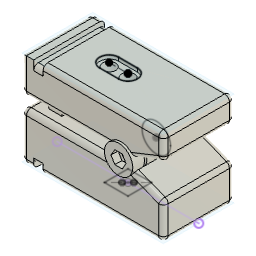
Pulse Oximeter v1 v4 (Autodesk Fusion 360 design; units mm, degrees)
Autodesk Fusion 360 part; units mm, degrees
sketch "Sketch1" plane through (0, 0, 0) normal (0, 0, 1) x (1, 0, 0)
  line L0 (30, 15) -> (-30, 15)
  line L1 (-30, 15) -> (-30, -15)
  line L2 (-30, -15) -> (30, -15)
  line L3 (30, -15) -> (30, 15)
  line L4 (30, 15) -> (-30, -15) construction
  line L5 (-30, 15) -> (30, -15) construction
  dimension "d1" = 30
  dimension "d2" = 60
  constraint horizontal L0
  constraint perpendicular L0 L1
  constraint parallel L0 L2
  constraint parallel L1 L3
  constraint coincident L4 origin
  constraint coincident L5 origin
  measures "d1" distance of L0 L2
  measures "d2" distance of L1 L3
extrude "Extrude1" add sketch "Sketch1" along normal blind 20 makes body 1
sketch "Sketch2" plane through (0, 0, 20) normal (0, 0, 1) x (-1, 0, 0)
  line L0 (-30, 15) -> (-30, -15)
  line L1 (-30, -15) -> (30, -15)
  line L2 (30, -15) -> (30, 15)
  line L3 (30, 15) -> (-30, 15)
  line L4 (30, -15) -> (-30, -15)
  line L5 (-30, -15) -> (-30, 15)
  line L6 (-30, 15) -> (30, 15)
  line L7 (30, 15) -> (30, -15)
  constraint horizontal L4
  constraint vertical L5
  constraint horizontal L6
  constraint vertical L7
  constraint coincident L0.start L3.end
  constraint coincident L1.end L2.start
extrude "Extrude2" add sketch "Sketch2" along normal blind 15 from surface at 5 separate body makes body 2
copy_body "Body->Comp1" bodies 2 removing the originals makes body 3 in component "Top"
sketch "Sketch3" plane through (0, 0, 0) normal (0, 1, 0) x (1, 0, 0)
  circle A0 centre (12, -22.5) radius 6
  line L0 (-30, 0) -> (30, 0)
  dimension "d8" = 12
  dimension "d9" = 12
  dimension "d10" = 22.5
  measures "d8" diameter of A0
  measures "d9" horizontal distance of origin A0.centre
  measures "d10" distance of A0.centre L0
move_face "MoveFace1" by (0, 0, 20) 1 faces at (10, 15, 30) on bodies 3 in component "Top"
move_body "Move1" bodies 1 to x (1, 0, 0) y (0, 1, 0) z (0, 0, 1) at (0, 0, -15)
extrude "Extrude1'" add sketch "Sketch3" along normal blind 5 from surface at 11 bodies 3 in component "Top"
extrude "Extrude2'" add sketch "Sketch3" along normal blind 5 from surface at -16 bodies 3 in component "Top"
sketch "Sketch4" plane through (0, 0, 0) normal (0, 1, 0) x (1, 0, 0)
  circle A0 centre (12, -7.5) radius 6
  line L0 (30, 15) -> (-30, 15)
  line L1 (30, 15) -> (30, -5)
  dimension "d17" = 12
  dimension "d19" = 22.5
  dimension "d20" = 18
  measures "d17" diameter of A0
  measures "d19" distance of A0.centre L0
  measures "d20" distance of A0.centre L1
extrude "Extrude3" add sketch "Sketch4" along normal mid plane 20 bodies 1
extrude "Extrude4" cut sketch "Sketch4" along normal through all from surface at 10 bodies 1
extrude "Extrude5" cut sketch "Sketch4" along normal up to surface (10 mm away) from surface at -20 bodies 1
move_body "Move2" bodies 1 to x (1, 0, 0) y (0, 1, 0) z (0, 0, 1) at (0, 0, 15)
sketch "Sketch5" plane through (0, 16, 0) normal (0, 1, 0) x (-1, 0, 0)
  circle A0 centre (-12, 22.5) radius 6
  circle A1 centre (-12, 22.5) radius 1.5
  dimension "d28" = 3
  constraint concentric A0 A1
  measures "d28" diameter of A1
extrude "Extrude6" cut sketch "Sketch5" against normal blind 39 contours A1 bodies 1
extrude "Extrude3'" cut sketch "Sketch5" against normal blind 39 contours A1 bodies 3 in component "Top"
sketch "Sketch6" plane through (0, 16, 0) normal (0, 1, 0) x (-1, 0, 0)
  circle A0 centre (-12, 22.5) radius 1.5
  circle A1 centre (-12, 22.5) radius 6
  circle A2 centre (-12, 22.5) radius 2.75
  dimension "d33" = 5.5
  constraint concentric A0 A2
  measures "d33" diameter of A2
extrude "Extrude4'" cut sketch "Sketch6" against normal blind 3 contours A2 bodies 3 in component "Top"
sketch "Sketch7" plane through (0, -16, 0) normal (0, -1, 0) x (1, 0, 0)
  circle A0 centre (12, 22.5) radius 1.5
  circle A1 centre (12, 22.5) radius 6
  line L0 (15.1754, 22.5) -> (13.5877, 25.25)
  line L1 (13.5877, 25.25) -> (10.4123, 25.25)
  line L2 (10.4123, 25.25) -> (8.8246, 22.5)
  line L3 (8.8246, 22.5) -> (10.4123, 19.75)
  line L4 (10.4123, 19.75) -> (13.5877, 19.75)
  line L5 (13.5877, 19.75) -> (15.1754, 22.5)
  point P0 (12, 22.5)
  dimension "d36" = 5.5
  constraint coincident P0 A0.centre
  constraint horizontal L4
  measures "d36" distance of L2 L5
extrude "Extrude5'" cut sketch "Sketch7" against normal blind 3 contours L0 L1 L2 L3 L4 L5 bodies 3 in component "Top"
sketch "Sketch8" plane through (0, 15, 0) normal (0, 1, 0) x (-1, 0, 0)
  arc A0 (-6.5456, 25) -> (-17.4544, 25) centre (-12, 22.5) ccw
  line L0 (-6.5456, 25) -> (30, 25)
  line L1 (30, 25) -> (30, 40)
  line L2 (30, 40) -> (-30, 40)
  line L3 (-30, 40) -> (-30, 25)
  line L4 (-30, 25) -> (-17.4544, 25)
  line L5 (-17.4544, 25) -> (-30, 25)
  line L6 (-30, 25) -> (-30, 30)
  line L7 (-30, 30) -> (-17.4544, 30) construction
  line L8 (-17.4544, 30) -> (-17.4544, 25) construction
  line L9 (-30, 30) -> (-17.4544, 25)
  line L10 (-12, 22.5) -> (-25, 22.5) construction
  line L11 (-12, 22.5) -> (-25, 22.5) construction
  line L12 (-30, 15) -> (-17.4544, 20)
  line L13 (-30, 20) -> (-30, 15)
  line L14 (-17.4544, 20) -> (-30, 20)
  dimension "d39" = 5
  constraint horizontal L5
  constraint vertical L6
  constraint horizontal L7
  constraint vertical L8
  constraint coincident L3 L6.end
  constraint coincident A0.end L4.end
  constraint coincident A0.centre L10.start
  constraint perpendicular L3 L10
  constraint symmetric A0.centre L10 L11.start
  constraint symmetric L11.end L10 L10.end
  constraint symmetric A0.end L10 L12.end
  constraint symmetric L3.end L10 L13.start
  constraint symmetric L6.end L10 L12.start
  measures "d39" distance of L5 L7
extrude "Extrude7" cut sketch "Sketch8" against normal blind 45 contours L3 L4 L5 L6 L9 | L12 L13 L14 bodies 1
extrude "Extrude6'" cut sketch "Sketch8" against normal blind 45 contours L3 L4 L5 L6 L9 | L12 L13 L14 bodies 3 in component "Top"
sketch "Sketch9" plane through (-30, 0, 0) normal (-1, 0, 0) x (0, -1, 0)
  line L0 (-15, 25) -> (15, 25)
  line L1 (15, 25) -> (15, 40)
  line L2 (15, 40) -> (-15, 40)
  line L3 (-15, 40) -> (-15, 25)
  circle A0 centre (0, 22.5) radius 8
  line L4 (-15, 0) -> (15, 0)
  line L5 (-15, 0) -> (-15, 20)
  dimension "d44" = 16
  dimension "d45" = 22.5
  dimension "d46" = 15
  measures "d44" diameter of A0
  measures "d45" distance of A0.centre L4
  measures "d46" distance of A0.centre L5
extrude "Extrude8" cut sketch "Sketch9" against normal blind 35 draft -2 contours L0 A0 | L0 A0 bodies 1
extrude "Extrude7'" cut sketch "Sketch9" against normal blind 35 draft -2 contours L0 A0 | L0 A0 bodies 3 in component "Top"
sketch "Sketch10" plane through (0, 0, 40) normal (0, 0, 1) x (-1, 0, 0)
  line L0 (30, 15) -> (-30, 15)
  line L1 (-30, 15) -> (-30, -15)
  line L2 (-30, -15) -> (30, -15)
  line L3 (30, -15) -> (30, 15)
  circle A0 centre (0, 0) radius 2.75
  circle A1 centre (8, 0) radius 2.75
  dimension "d55" = 30
  dimension "d56" = 5.5
  dimension "d57" = 8
  dimension "d58" = 5.5
  dimension "d59" = 15
  dimension "d60" = 15
  measures "d55" distance of L3 A0.centre
  measures "d56" diameter of A0
  measures "d57" distance of A0.centre A1.centre
  measures "d58" diameter of A1
  measures "d59" distance of L2 A1.centre
  measures "d60" distance of L2 A0.centre
extrude "Extrude9" cut sketch "Sketch10" against normal blind 60 contours A0 | A1 bodies 1
extrude "Extrude8'" cut sketch "Sketch10" against normal blind 60 contours A0 | A1 bodies 3 in component "Top"
sketch "Sketch12" plane through (0, 0, 40) normal (0, 0, 1) x (-1, 0, 0)
  circle A0 centre (0, 0) radius 2.75
  circle A1 centre (8, 0) radius 2.75
  line L0 (30, 15) -> (-30, 15)
  line L1 (-30, 15) -> (-30, -15)
  line L2 (-30, -15) -> (30, -15)
  line L3 (30, -15) -> (30, 15)
  line L4 (0, -4) -> (8, -4)
  arc A2 (8, -4) -> (8, 4) centre (8, 0) ccw
  line L5 (8, 4) -> (0, 4)
  arc A3 (0, 4) -> (0, -4) centre (0, 0) ccw
  line L6 (0, 0) -> (8, 0) construction
  dimension "d65" = 8
  constraint tangent L4 A2
  constraint tangent A2 L5
  constraint parallel L4 L5
  constraint tangent L5 A3
  constraint tangent L4 A3
  constraint coincident A1.centre A2.centre
  constraint horizontal L6
  constraint coincident A0.centre A3.centre
  measures "d65" distance of L4 L5
extrude "Extrude9'" cut sketch "Sketch12" against normal blind 1.5 contours L4 A2 L5 A3 bodies 3 in component "Top"
sketch "Sketch13" plane through (0, 0, 0) normal (0, 0, -1) x (1, 0, 0)
  circle A0 centre (0, 0) radius 2.75 construction
  circle A1 centre (-8, 0) radius 2.75
  line L0 (30, -15) -> (30, 15)
  line L1 (30, 15) -> (-30, 15)
  line L2 (-30, 15) -> (-30, -15)
  line L3 (-30, -15) -> (30, -15)
  line L4 (5, -5) -> (-5, -5)
  line L5 (-5, -5) -> (-5, 5)
  line L6 (-5, 5) -> (5, 5)
  line L7 (5, 5) -> (5, -5)
  line L8 (5, -5) -> (-5, 5) construction
  circle A2 centre (1.2374, -1.2374) radius 1
  circle A3 centre (-1.2374, 1.2374) radius 1
  dimension "d68" = 10
  dimension "d69" = 10
  dimension "d70" = 10
  dimension "d71" = 25
  dimension "d72" = 2
  dimension "d73" = 2
  constraint horizontal L4
  constraint vertical L5
  constraint horizontal L6
  constraint vertical L7
  constraint coincident L8 A2.centre
  constraint coincident L8 A3.centre
  constraint tangent A0 A3
  constraint tangent A0 A2
  measures "d68" distance of L3 L4
  measures "d69" distance of L5 L7
  measures "d70" distance of L4 L6
  measures "d71" distance of L2 L5
  measures "d72" diameter of A2
  measures "d73" diameter of A3
extrude "Extrude10" add sketch "Sketch13" against normal blind 13 contours L4 L5 L6 L7 bodies 1
sketch "Sketch14" plane through (0, 15, 0) normal (0, 1, 0) x (-1, 0, 0)
  line L0 (-30, 30) -> (-17.4544, 25)
  arc A0 (-6.5456, 25) -> (-17.4544, 25) centre (-12, 22.5) ccw
  line L1 (-6.5456, 25) -> (30, 25)
  line L2 (30, 25) -> (30, 40)
  line L3 (30, 40) -> (-30, 40)
  line L4 (-30, 40) -> (-30, 30)
  line L5 (21, 40) -> (25, 40)
  line L6 (25, 40) -> (25, 38)
  line L7 (25, 38) -> (21, 38)
  line L8 (21, 38) -> (21, 40)
  line L9 (21, 0) -> (25, 0)
  line L10 (25, 0) -> (25, 2)
  line L11 (25, 2) -> (21, 2)
  line L12 (21, 2) -> (21, 0)
  line L13 (30, 0) -> (-30, 0)
  line L14 (30, 0) -> (30, 20)
  dimension "d76" = 2
  dimension "d77" = 4
  dimension "d78" = 5
  dimension "d79" = 2
  dimension "d80" = 4
  dimension "d81" = 5
  constraint horizontal L5
  constraint vertical L6
  constraint horizontal L7
  constraint vertical L8
  constraint coincident L3 L5.start
  constraint horizontal L9
  constraint vertical L10
  constraint horizontal L11
  constraint vertical L12
  constraint coincident L9.start L13
  measures "d76" distance of L5 L7
  measures "d77" distance of L6 L8
  measures "d78" distance of L2 L6
  measures "d79" distance of L9 L11
  measures "d80" distance of L10 L12
  measures "d81" distance of L10 L14
extrude "Extrude11" cut sketch "Sketch14" against normal up to surface (30 mm away) contours L3 L5 L6 L7 L8 | L9 L10 L11 L12 L13 bodies 1
extrude "Extrude10'" cut sketch "Sketch14" against normal up to surface (30 mm away) contours L3 L5 L6 L7 L8 | L9 L10 L11 L12 L13 bodies 3 in component "Top"
extrude "Extrude12" cut sketch "Sketch12" along normal blind 7 from surface at -40 contours A0 | L4 A2 L5 A3 bodies 1
fillet "Fillet1" radius 2 18 edges at (4.5, -15, 0) (-30, -15, 10) (-11.7272, -15, 20) (23.7272, -15, 17.5) (30, 0, 0) (30, 0, 15) (-27.5, -15, 0) (-23, -15, 2) (-30, 0, 0) (-30, 15, 10) (-11.7272, 15, 20) (4.5, 15, 0) (-23, 15, 2) (-27.5, 15, 0) (30, 15, 7.5) (23.7272, 15, 17.5) (-30, 11.2997, 20) (-30, -11.2997, 20) on bodies 1
fillet "Fillet1" radius 2 1 edges at (30, -15, 7.5) on bodies 1
fillet "Fillet1'" radius 2 17 edges at (-11.7272, -15, 25) (-30, -15, 32.5) (4.5, -15, 40) (30, -15, 35) (23.7272, -15, 27.5) (30, 0, 40) (30, 0, 30) (23.7272, 15, 27.5) (30, 15, 35) (4.5, 15, 40) (-23, 15, 38) (-27.5, 15, 40) (-30, 15, 32.5) (-11.7272, 15, 25) (-30, 11.2997, 25) (-30, -11.2997, 25) (-30, 0, 40) on bodies 3 in component "Top"
fillet "Fillet1'" radius 2 1 edges at (-23, -15, 38) on bodies 3 in component "Top"
sketch "Sketch15" plane through (0, 0, 25) normal (0, 0, -1) x (1, 0, 0)
  line L0 (-28, -7.5258) -> (-28, -13)
  line L1 (-28, -13) -> (6.5456, -13)
  line L2 (6.5456, -13) -> (6.5456, -11)
  line L3 (6.5456, -11) -> (17.4544, -11)
  line L4 (17.4544, -11) -> (17.4544, 11)
  line L5 (17.4544, 11) -> (6.5456, 11)
  line L6 (6.5456, 11) -> (6.5456, 13)
  line L7 (6.5456, 13) -> (-28, 13)
  line L8 (-28, 13) -> (-28, 7.5258)
  spline S0 degree 2 poles (-28, 7.5258) (-10.0369, 6.8648) (5, 6.2999) knots 0.183241 0.183241 0.183241 3.502412 3.502412 3.502412 weights 1.000386 1.003685 1
  line L9 (5, 6.2999) -> (5, -6.2999)
  spline S1 degree 2 poles (5, -6.2999) (-10.0369, -6.8648) (-28, -7.5258) knots 0 0 0 3.319171 3.319171 3.319171 weights 1 1.003685 1.000386
  line L10 (-22, 12) -> (-16, 12)
  line L11 (-16, 12) -> (-16, 9)
  line L12 (-16, 9) -> (-22, 9)
  line L13 (-22, 9) -> (-22, 12)
  line L14 (-30, 0) -> (30, 0)
  line L15 (-22, -12) -> (-16, -12)
  line L16 (-16, -12) -> (-16, -9)
  line L17 (-22, -9) -> (-22, -12)
  line L18 (-16, -9) -> (-22, -9)
  dimension "d91" = 3
  dimension "d92" = 6
  dimension "d93" = 6
  dimension "d94" = 1
  constraint horizontal L10
  constraint vertical L11
  constraint horizontal L12
  constraint vertical L13
  constraint symmetric L10.start L14 L15.start
  constraint symmetric L10.end L14 L15.end
  constraint symmetric L11.end L14 L16.end
  constraint symmetric L12.end L14 L17.start
  measures "d91" distance of L10 L12
  measures "d92" distance of L11 L13
  measures "d93" distance of L8 L13
  measures "d94" distance of L7 L10
extrude "Extrude11'" add sketch "Sketch15" along normal blind 3 draft -5 contours L10 L11 L12 L13 | L15 L16 L17 L18 bodies 3 in component "Top"
fillet "Fillet2" radius 1 8 edges at (-19, -12, 25) (-22, -10.5, 25) (-19, -9, 25) (-16, -10.5, 25) (-22, 10.5, 25) (-19, 12, 25) (-16, 10.5, 25) (-19, 9, 25) on bodies 3 in component "Top"
component "Top" placed x (1, 0, 0) y (0, 1, 0) z (0, 0, 1) at (0, 0, 0)
